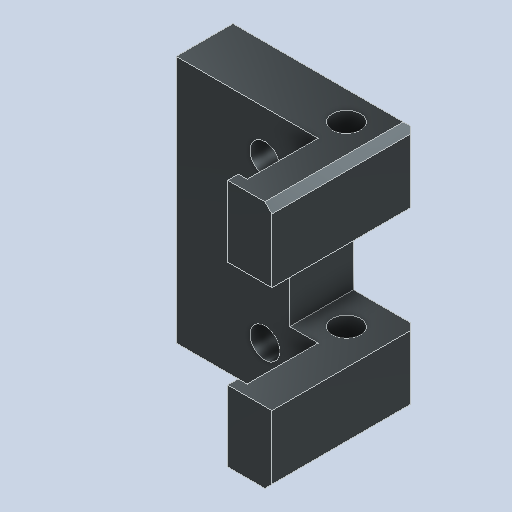
# Autodesk Inventor part: Lager
Saved by Autodesk Inventor 2023.2 (Build 272271030, 271C)
## iProperties
Created: 2023-02-12
Part Number: Lager
Material: Iron, Cast
Document SubType Name: Modeling
Designer: Ayush
Density: 7.15 g/cm^3
Appearance: Iron Gray
Author: Ayush
Autodesk Inventor part; units mm, degrees
ref_plane "YZ Plane" through (0, 0, 0) normal (1, 0, 0) x (0, 1, 0)
sketch "Sketch1" plane through (0, 0, 0) normal (0, 1, 0) x (-1, 0, 0)
  line L0 (0, -20) -> (40, -20)
  line L1 (40, -20) -> (40, -38)
  line L2 (0, -20) -> (0, 0)
  line L3 (0, 0) -> (2.5, 0)
  line L4 (2.5, 0) -> (2.5, 3)
  line L5 (2.5, 3) -> (-10, 3)
  line L6 (-10, 3) -> (-10, -38)
  line L7 (-10, -38) -> (40, -38)
  circle A0 centre (0, -28) radius 4
  point P0 (-3.75, 3)
  point P1 (1.25, 0)
  dimension "d1" = 40
  dimension "d2" = 18
  dimension "d4" = 12.5
  dimension "d5" = 10
  dimension "d6" = 3
  dimension "d7" = 20
  dimension "d8" = 8
  dimension "d9" = 10
  dimension "d10" = 10
  constraints: 16 end point, 4 perpendicular, 2 midpoint, 2 vertical, 1 centre point, 1 horizontal
  measures "d1" distance of L0.start L0.end
  measures "d2" distance of L0.end L1.end
  measures "d4" distance of L4.end L5.end
  measures "d5" distance between parallel lines of L6 L2
  measures "d6" vertical distance of point (-3.75, 3) point (1.25, 0)
  measures "d7" distance of L0.start L2.end
  measures "d8" diameter of A0
  measures "d9" distance from line of L6 A0.centre
  measures "d10" distance from line of L7 A0.centre
extrude "Extrusion1" add sketch "Sketch1" along normal blind 20
sketch "Sketch2" plane through (0, 0, 0) normal (0, -1, 0) x (1, 0, 0)
  point P0 (0, 0)
sketch "Sketch3" plane through (0, 0, 0) normal (0, -1, 0) x (1, 0, 0)
  line L0 (10, -38) -> (-40, -38) projected
  line L1 (-8, -38) -> (-8, -20)
  line L2 (-40, -20) -> (0, -20) projected
  line L3 (10, 3) -> (10, -38) projected
  line L4 (-8, -38) -> (-40, -38)
  line L5 (-40, -38) -> (-40, -20) projected
  line L6 (-40, -20) -> (-8, -20)
  point P0 (0, 0)
  dimension "d13" = 18
  constraints: 6 end point, 2 point on line, 1 collinear, 1 parallel, 1 vertical
  measures "d13" distance between parallel lines of L1 L3
extrude "Extrusion2" add sketch "Sketch3" along normal blind 15
ref_plane "Work Plane1" through (0, -15, 0) normal (0, -1, 0) x (1, 0, 0)
mirror "Mirror1" about plane through (0, -15, 0) normal (0, -1, 0) of "Extrusion1"
ref_plane "Work Plane2" through (0, -15, 0) normal (0, -1, 0) x (1, 0, 0)
mirror "Mirror2" about plane through (0, -15, 0) normal (0, -1, 0) of "Extrusion2"
sketch "Sketch4" plane through (10, 20, -38) normal (0, 0, -1) x (-1, 0, 0)
  circle A0 centre (25, -12.5) radius 7.5
  circle A1 centre (25, -57.5) radius 7.5
  line L0 (50, -70) -> (50, 0) projected
  line L1 (0, 0) -> (50, 0) projected
  line L2 (0, -70) -> (50, -70) projected
  point P0 (10, -20)
  dimension "d18" = 15
  dimension "d19" = 15
  dimension "d20" = 25
  dimension "d21" = 12.5
  dimension "d22" = 12.5
  dimension "d23" = 25
  constraints: 2 centre point
  measures "d18" diameter of A0
  measures "d19" diameter of A1
  measures "d20" distance from line of A0.centre L0
  measures "d21" distance from line of L1 A0.centre
  measures "d22" distance from line of L2 A1.centre
  measures "d23" distance from line of A1.centre L0
hole "Hole1" at (-15, 7.5, -38) at (-15, -37.5, -38) direction (0, 0, 1) diameter 15 depth 8 tip angle 118
sketch "Sketch5" plane through (10, 20, -38) normal (0, 0, -1) x (-1, 0, 0)
  circle A0 centre (25, -12.5) radius 4.2
  circle A1 centre (25, -57.5) radius 4.2
  line L0 (50, -70) -> (50, 0) projected
  line L1 (0, 0) -> (50, 0) projected
  line L2 (0, -70) -> (50, -70) projected
  point P0 (10, -20)
  dimension "d31" = 8.4
  dimension "d32" = 8.4
  dimension "d33" = 25
  dimension "d34" = 12.5
  dimension "d35" = 25
  dimension "d36" = 12.5
  constraints: 2 centre point
  measures "d31" diameter of A0
  measures "d32" diameter of A1
  measures "d33" distance from line of A0.centre L0
  measures "d34" distance from line of A0.centre L1
  measures "d35" distance from line of A1.centre L0
  measures "d36" distance from line of L2 A1.centre
hole "Hole2" at (-15, 7.5, -38) at (-15, -37.5, -38) direction (0, 0, 1) diameter 8.4 end through all
chamfer "Chamfer1" distance 2 angle 45 1 edges at (-15, 20, -38) measured on face at (-33.7241, -8.9202, -38)
chamfer "Chamfer2" distance 2 angle 45 1 edges at (-40, -16, -38) measured on face at (-33.7241, -21.7465, -38)
chamfer "Chamfer3" distance 2 angle 45 1 edges at (-14, -50, -38) measured on face at (-32.3908, -21.7465, -38)
chamfer "Chamfer4" distance 2 angle 45 1 edges at (10, 9, -38) measured on face at (-32.3908, -21.0798, -38)
chamfer "Chamfer5" distance 2 angle 45 1 edges at (10, -39, -38) measured on face at (-32.3908, -21.0798, -38)
chamfer "Chamfer6" distance 2 angle 45 1 edges at (10, 20, -16.5) measured on face at (-28, 20, -28)
chamfer "Chamfer7" distance 2 angle 45 1 edges at (10, -50, -16.5) measured on face at (-28, -50, -28)
body "Solid1"
